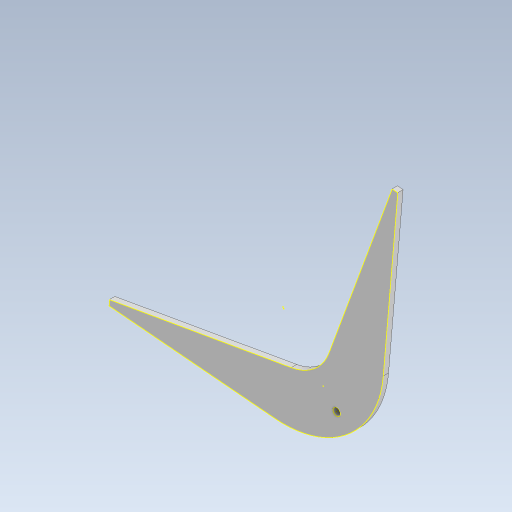
# Autodesk Inventor part: sus_2
Saved by Autodesk Inventor 2023 (Build 270158000, 158)
## iProperties
Created: 2023-06-07
Part Number: sus_2
Material: 一般
Document SubType Name: Modeling
Designer: JOU
Density: 1 g/cm^3
Appearance: 預設
Author: JOU
Autodesk Inventor part; units mm, degrees
ref_plane "YZ Plane" through (0, 0, 0) normal (1, 0, 0) x (0, 1, 0)
ref_plane "XZ Plane" through (0, 0, 0) normal (0, 1, 0) x (-1, 0, 0)
ref_plane "XY Plane" through (0, 0, 0) normal (0, 0, 1) x (1, 0, 0)
sketch "草圖1" plane through (0, 0, 0) normal (0, 0, 1) x (1, 0, 0)
  arc A0 (-17.0574, -3.0077) -> (5.924, 16.276) centre (-22.2668, 26.5366) ccw
  line L0 (5.924, 16.276) -> (41.0424, 112.7631)
  line L1 (-118.1769, -20.8378) -> (-17.0574, -3.0077)
  line L2 (-118.1769, -20.8378) -> (-26.5575, -28.8534)
  arc A1 (-26.5575, -28.8534) -> (33.0268, 21.1437) centre (-21.764, 25.9373) ccw
  line L3 (33.0268, 21.1437) -> (41.0424, 112.7631)
  circle A2 centre (7.3253, -8.7299) radius 2
  arc A3 (-17.5783, -0.0533) -> (3.1049, 17.302) centre (-22.2668, 26.5366) ccw
  line L4 (3.1049, 17.302) -> (46.017, 135.2022)
  line L5 (46.017, 135.2022) -> (36.0153, 20.8822)
  arc A4 (-26.819, -31.842) -> (36.0153, 20.8822) centre (-21.764, 25.9373) ccw
  line L6 (-26.819, -31.842) -> (-141.1389, -21.8403)
  line L7 (-141.1389, -21.8403) -> (-17.5783, -0.0533)
  line L8 (41.0424, 112.7631) -> (37.9484, 113.0338)
  line L9 (-118.1769, -20.8378) -> (-117.9062, -17.7438)
  point P0 (0, 0)
  dimension "d0" = 55
  dimension "d1" = 4
  dimension "d2" = 23
  dimension "d3" = 23
  dimension "d6" = 3
  constraints: 20 end point, 8 point on circle, 5 centre point, 5 perpendicular, 2 point on line, 2 tangent, 13 other
  measures "d0" radius of A1
  measures "d1" diameter of A2
  measures "d2" distance from line of L3 A2.centre
  measures "d3" distance from line of L2 A2.centre
  measures "d6" distance between parallel lines of L1 L7
extrude "擠出1" add sketch "草圖1" along normal blind 3 contours L1 L9 L7 A3 L4 L8 L0 A0 | A0 L0 L3 A1 L2 L1
sketch "草圖2" plane through (0, 0, 3) normal (0, 0, 1) x (1, 0, 0)
  arc A0 (-26.5575, -28.8534) -> (33.0268, 21.1437) centre (-21.764, 25.9373) ccw projected
  line L0 (33.0268, 21.1437) -> (41.0424, 112.7631) projected
  line L1 (41.0424, 112.7631) -> (37.9484, 113.0338) projected
  line L2 (37.9484, 113.0338) -> (3.1049, 17.302) projected
  arc A1 (-17.5783, -0.0533) -> (3.1049, 17.302) centre (-22.2668, 26.5366) ccw projected
  line L3 (-17.5783, -0.0533) -> (-117.9062, -17.7438) projected
  line L4 (-117.9062, -17.7438) -> (-118.1769, -20.8378) projected
  line L5 (-118.1769, -20.8378) -> (-26.5575, -28.8534) projected
  circle A2 centre (7.3253, -8.7299) radius 2 projected
  point P0 (0, 0)
equation "\"d3\" = d2"
